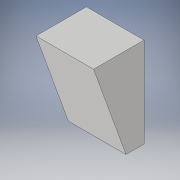
# Autodesk Inventor part: BT100_trajan20_21
Saved by Autodesk Inventor 2022.2 (Build 262287000, 287)
## iProperties
Company: HTBLA Kaindorf
RuleStatus: InUse
Created: 2022-09-27
Part Number: BT100_trajan20_21
Project: Zeichenmaschine_v2_a
Material: Generisch
Description: uniblock_3dDruck
Document SubType Name: Modeling
Designer: trajan20
Density: 1 g/cm^3
Appearance: Vorgabe
Mass: 3.8 g
Surface Area: 16.0413 cm^2
Volume: 3.8 cm^3
AfterDocNew0: iProperties-Editor_aufrufen
Author: jan
Keywords: 2021
Autodesk Inventor part; units mm, degrees
note: some values were not read from the file. Chosen so that the rebuilt part matches the saved one: second side of "Extrusion3".
ref_plane "YZ Plane" through (0, 0, 0) normal (1, 0, 0) x (0, 1, 0)
ref_plane "XZ Plane" through (0, 0, 0) normal (0, 1, 0) x (-1, 0, 0)
ref_plane "XY Plane" through (0, 0, 0) normal (0, 0, 1) x (1, 0, 0)
sketch "Skizze3" plane through (0, 0, 0) normal (0, 1, 0) x (-1, 0, 0)
  line L0 (0, 0) -> (14, 0)
  line L1 (14, 0) -> (14, -25)
  line L2 (14, -25) -> (9, -25)
  line L3 (9, -25) -> (0, 0)
  dimension "d4" = 25
  dimension "d5" = 14
  dimension "d6" = 5
  constraints: 8 end point, 2 perpendicular, 1 horizontal
  measures "d4" distance between parallel lines of L2 L0
  measures "d5" distance from line of L1 L0.start
  measures "d6" distance from line of L2.end L1
extrude "Extrusion3" add sketch "Skizze3" along normal blind 16
